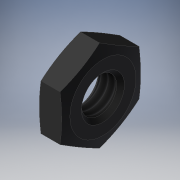
# Autodesk Inventor part: ISO 4035 M3(F)
Saved by Autodesk Inventor 2019 (Build 230136000, 136)
## iProperties
Created: 2024-05-27
Part Number: ISO 4035 M3(F)
Material: Generic
Catalog Web Link: www.cadenas.de
Description: ISO 4035-Hexagon thin nuts (chamfered) - Product grades A and B
Vendor: FESTO
Document SubType Name: Modeling
Designer: psAdmin
Manufacturer: FESTO
Mass: 0.0363579 g
Surface Area: 0.834298 cm^2
Volume: 0.0363579 cm^3
Density: 1 g/cm^3
Appearance: PSOLRGB-175-175-175
Category: PARTsolutions
Company: FESTO
Title: ISO 4035 M3(F)
Author: Cadenas PARTsolutions
Comments: Hexagon thin nuts (chamfered) - Product grades A and B
PSOL_IDENT_0: {$CADENAS_DATA/23d-libs/festo/zyl_zubeh/iso_4035/din_iso_4035.prj},170 {VTYP=3D},{NB=ISO 4035 M3(F)}
PSOL_IDENT_1: ,{LINA=ISO 4035 M3(F)},{NN=ISO 4035},{DATE=13.09.2023 12:11:15},{GEOMDATE=13.09.2023 12:10:57},{VERS
PSOL_IDENT_2: ION=},{LINEID=40},{WBVAR=},{WBNUMERIC=}  {NB=ISO 4035 M3(F)},{LINA=ISO 4035 M3(F)},{KT=X},{IDNR=},{N
PSOL_IDENT_3: ENN=M3},{D=3.000},{D1=2.459},{P=0.500},{D2=4.600},{E=6.010},{M=1.800},{S=5.500},{CNSAVOID=0},{DIST=0
PSOL_IDENT_4: .223143}
NB: ISO 4035 M3(F)
NN: ISO 4035
NT: Hexagon thin nuts (chamfered) - Product grades A and B
NBSYN: ISO 4035 $NENN.(F)
LINA: ISO 4035 M3(F)
CATALOG: Festo
ROWDESC: M3
NENN: M3
D: 3
D1: 2.459
P: 0.5
D2: 4.6
E: 6.01
M: 1.8
S: 5.5
SUPPLIER: FESTO
ARTICLENO: ISO 4035 M3(F)
BOMINFO: ISO 4035 M3(F)
CREATOR: CADENAS GmbH
Autodesk Inventor part; units mm, degrees
sketch "Sketch_1" plane through (0, 0, 0) normal (0, 1, 0) x (-1, 0, 0)
  line L0 (-1.8, 0) -> (0, 0)
  line L1 (0, 0) -> (0, -3.3)
  line L2 (0, -3.3) -> (-1.8, -3.3)
  line L3 (-1.8, -3.3) -> (-1.8, 0)
  line L4 (-1.8, 0) -> (0, 0)
  constraints: 10 end point
revolve "Revolution1" add sketch "Sketch_1" angle 360 about axis through (1.8, 0, 0) along (1, 0, 0)
sketch "Sketch_3" plane through (0, 0, 0) normal (0, 0, 1) x (1, 0, 0)
  line L0 (1.8, 0) -> (0, 0)
  line L1 (-2.3, 5.5) -> (-2.3, 2.3)
  line L2 (-2.3, 2.3) -> (0, 2.3)
  line L3 (0, 2.3) -> (0.2679, 3.3)
  line L4 (0.2679, 3.3) -> (1.5321, 3.3)
  line L5 (1.5321, 3.3) -> (1.8, 2.3)
  line L6 (1.8, 2.3) -> (4.1, 2.3)
  line L7 (4.1, 2.3) -> (4.1, 5.5)
  line L8 (4.1, 5.5) -> (-2.3, 5.5)
  constraints: 18 end point
revolve "Revolution2" cut sketch "Sketch_3" angle 360 about axis through (1.8, 0, 0) along (1, 0, 0)
sketch "Skizze_3" plane through (0, 0, 0) normal (0, 0, 1) x (1, 0, 0)
  line L0 (1.8, 0) -> (0, 0)
  line L1 (0, 0) -> (0, 1.5)
  line L2 (0, 1.5) -> (0.2705, 1.2295)
  line L3 (0.2705, 1.2295) -> (1.5295, 1.2295)
  line L4 (1.5295, 1.2295) -> (1.8, 1.5)
  line L5 (1.8, 1.5) -> (1.8, 0)
  line L6 (1.8, 0) -> (0, 0)
  constraints: 14 end point
revolve "Revolution3" cut sketch "Skizze_3" angle 360 about axis through (1.8, 0, 0) along (1, 0, 0)
thread "Thread1" size "M3x0.5" class "6H" standard "ISO Metric profile" full length
sketch "Sketch_2" plane through (0, 0, 0) normal (1, 0, 0) x (0, 1, 0)
  line L0 (11, 11) -> (-11, 11)
  line L1 (-11, 11) -> (-11, -11)
  line L2 (-11, -11) -> (11, -11)
  line L3 (11, -11) -> (11, 11)
  line L4 (1.5877, 2.75) -> (-1.5877, 2.75)
  line L5 (-1.5877, 2.75) -> (-3.1754, 0)
  line L6 (-3.1754, 0) -> (-1.5877, -2.75)
  line L7 (-1.5877, -2.75) -> (1.5877, -2.75)
  line L8 (1.5877, -2.75) -> (3.1754, 0)
  line L9 (3.1754, 0) -> (1.5877, 2.75)
  constraints: 20 end point
extrude "Extrusion1" cut sketch "Sketch_2" along normal mid plane 5.6
ref_plane "2CYL_XY" through (0.9, 0, 0) normal (1, 0, 0) x (0, 0, -1)
ref_plane "2CYL_YZ" through (0.9, 0, 0) normal (0, 0, -1) x (0, 1, 0)
ref_plane "2CYL_ZX" through (0.9, 0, 0) normal (0, 1, 0) x (1, 0, 0)
ref_plane "IP1_XY" through (0, 0, 0) normal (1, 0, 0) x (0, 0, -1)
ref_plane "IP1_YZ" through (0, 0, 0) normal (0, 0, -1) x (0, 1, 0)
ref_plane "IP1_ZX" through (0, 0, 0) normal (0, 1, 0) x (1, 0, 0)
ref_plane "IP2_XY" through (1.8, 0, 0) normal (1, 0, 0) x (0, 0, -1)
ref_plane "IP2_YZ" through (1.8, 0, 0) normal (0, 0, -1) x (0, 1, 0)
ref_plane "IP2_ZX" through (1.8, 0, 0) normal (0, 1, 0) x (1, 0, 0)
body "Solid1"
